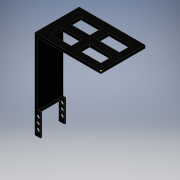
# Autodesk Inventor part: GrapperRight
Saved by Autodesk Inventor 2016 (Build 200138000, 138)
## iProperties
Created: 2016-03-30
Part Number: GrapperRight
Material: UHMW, Black
Document SubType Name: Modeling
Designer: mkepler
Density: 0.94 g/cm^3
Appearance: Smooth - Black
Mass: 11.6359 g
Surface Area: 108.063 cm^2
Volume: 12.3787 cm^3
Author: mkepler
Autodesk Inventor part; units mm, degrees
ref_plane "YZ Plane" through (0, 0, 0) normal (1, 0, 0) x (0, 1, 0)
ref_plane "XZ Plane" through (0, 0, 0) normal (0, 1, 0) x (-1, 0, 0)
ref_plane "XY Plane" through (0, 0, 0) normal (0, 0, 1) x (1, 0, 0)
sketch "Sketch3" plane through (0, 0, 0) normal (0, 1, 0) x (-1, 0, 0)
  line L0 (0, 0) -> (70, 0)
  line L1 (70, 0) -> (70, -70)
  line L2 (70, -70) -> (70, -94)
  line L3 (70, -94) -> (64, -94)
  line L4 (64, -94) -> (64, -70)
  line L5 (64, -3) -> (0, -3)
  line L6 (0, -3) -> (0, 0)
  line L7 (64, -70) -> (67, -70)
  line L8 (67, -70) -> (67, -3)
  line L9 (67, -3) -> (64, -3)
  circle A0 centre (67, -82) radius 2.125
  circle A1 centre (67, -76) radius 2.125
  circle A2 centre (67, -88) radius 2.125
  dimension "d26" = 70
  dimension "d27" = 70
  dimension "d29" = 6
  dimension "d55" = 4.25
  dimension "d56" = 4.25
  dimension "d57" = 4.25
  dimension "d59" = 6
  dimension "d60" = 6
  dimension "d61" = 6
  constraints: 20 end point, 6 perpendicular, 3 centre point, 2 horizontal, 2 point on line, 1 parallel
  measures "d26" distance of L0.start L0.end
  measures "d27" distance of L0.end L1.end
  measures "d29" distance of L2.end L3.end
  measures "d55" diameter of A0
  measures "d56" diameter of A1
  measures "d57" diameter of A2
  measures "d59" distance of A0.centre A2.centre
  measures "d60" distance from line of L7 A1.centre
  measures "d61" distance of A0.centre A1.centre
extrude "Extrusion2" add sketch "Sketch3" along normal blind 27 contours L0 L1 L2 L3 L4 L7 L8 L9 L5 L6 | A0 | A1 | A2
sketch "Sketch4" plane through (0, 27, 0) normal (0, 1, 0) x (1, 0, 0)
  line L0 (-70, 0) -> (0, 0) projected
  line L1 (0, 0) -> (0, 3) projected
  line L2 (-70, 0) -> (0, 0)
  line L3 (0, 0) -> (0, 3)
  line L4 (0, 3) -> (-70, 3)
  line L5 (-70, 3) -> (-70, 0)
  constraints: 8 end point, 2 parallel, 1 horizontal, 1 perpendicular
extrude "Extrusion3" add sketch "Sketch4" along normal blind 20
sketch "Sketch5" plane through (-70, 0, -94) normal (-1, 0, 0) x (0, 0, 1)
  line L0 (-0.1204, 1.5) -> (23.8796, 1.5)
  line L1 (23.8796, 1.5) -> (23.8796, 25.5)
  line L2 (23.8796, 25.5) -> (-0.1204, 25.5)
  line L3 (-0.1204, 25.5) -> (-0.1204, 1.5)
  line L4 (94, 0) -> (0, 0) projected
  dimension "d36" = 24
  dimension "d37" = 24
  dimension "d38" = 1.5
  constraints: 8 end point, 2 parallel, 1 horizontal, 1 perpendicular
  measures "d36" distance of L2.end L1.end
  measures "d37" distance of L1.end L0.end
  measures "d38" distance between parallel lines of L0 L4
extrude "Extrusion4" cut sketch "Sketch5" against normal blind 10
sketch "Sketch9" plane through (0, 0, -3) normal (0, 0, -1) x (-1, 0, 0)
  line L0 (7, 7) -> (60, 7)
  line L1 (60, 7) -> (60, 39)
  line L2 (60, 39) -> (7, 39)
  line L3 (7, 39) -> (7, 7)
  line L4 (0, 0) -> (0, 47) projected
  line L5 (67, 0) -> (0, 0) projected
  dimension "d45" = 53
  dimension "d46" = 32
  dimension "d47" = 7
  dimension "d48" = 7
  constraints: 8 end point, 2 parallel, 1 horizontal, 1 perpendicular
  measures "d45" distance of L2.end L1.end
  measures "d46" distance of L1.end L0.end
  measures "d47" distance between parallel lines of L4 L3
  measures "d48" distance between parallel lines of L5 L0
extrude "Extrusion5" cut sketch "Sketch9" against normal blind 10
sketch "Sketch10" plane through (-70, 0, 0) normal (0, 0, 1) x (1, 0, 0)
  line L0 (10, 39) -> (10, 7) projected
  line L1 (63, 7) -> (63, 39) projected
  line L2 (63, 26.6385) -> (63, 18.6385)
  line L3 (10, 18.6385) -> (10, 26.6385)
  line L4 (63, 39) -> (10, 39) projected
  line L5 (10, 7) -> (63, 7) projected
  line L6 (31.6097, 39) -> (39.6097, 39)
  line L7 (39.6097, 39) -> (39.6097, 7)
  line L8 (39.6097, 7) -> (31.6097, 7)
  line L9 (31.6097, 7) -> (31.6097, 18.6385)
  line L10 (31.6097, 26.6385) -> (31.6097, 39)
  line L11 (10, 26.6385) -> (31.6097, 26.6385)
  line L12 (39.6097, 26.6385) -> (63, 26.6385)
  line L13 (63, 18.6385) -> (39.6097, 18.6385)
  line L14 (31.6097, 18.6385) -> (10, 18.6385)
  point P0 (70, 0)
  dimension "d51" = 8
  dimension "d52" = 8
  constraints: 22 end point, 8 parallel, 6 point on line, 3 horizontal, 3 perpendicular
  measures "d51" distance of L2.start L2.end
  measures "d52" distance of L7.end L8.end
extrude "Extrusion6" add sketch "Sketch10" against normal blind 3 contours L11 L10 L4 L7 L5 L9 L14 L0 | L12 L1 L13 L7
sketch "Sketch11" plane through (0, 0, 0) normal (0, -1, 0) x (1, 0, 0)
  point P0 (0, 0)
sketch "Sketch12" plane through (0, 0, 0) normal (0, -1, 0) x (1, 0, 0)
  circle A0 centre (-67, -82) radius 2.125
  circle A1 centre (-67, -76) radius 2.125
  circle A2 centre (-67, -88) radius 2.125
  line L0 (-64, -70) -> (-67, -70) projected
  point P0 (0, 0)
  dimension "d62" = 4.25
  dimension "d63" = 4.25
  dimension "d64" = 4.25
  dimension "d65" = 6
  dimension "d66" = 6
  dimension "d67" = 6
  constraints: 3 centre point
  measures "d62" diameter of A0
  measures "d63" diameter of A1
  measures "d64" diameter of A2
  measures "d65" distance from line of L0 A1.centre
  measures "d66" distance of A0.centre A2.centre
  measures "d67" distance of A1.centre A0.centre
hole "Hole2" at (-67, 0, -88) at (-67, 0, -82) at (-67, 0, -76) direction (0, 1, 0) diameter 4.25 end through all
body "Solid2"
